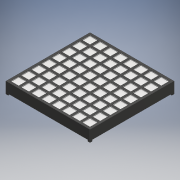
# Autodesk Inventor part: Pieza1
Saved by Autodesk Inventor 2017 (Build 210142000, 142)
## iProperties
Part Number: Pieza1
Material: Genérico
Document SubType Name: Modeling
Designer: Roberto
Density: 1 g/cm^3
Appearance: Valor por defecto
Author: Roberto
Autodesk Inventor part; units mm, degrees
ref_plane "YZ Plane" through (0, 0, 0) normal (1, 0, 0) x (0, 1, 0)
ref_plane "XZ Plane" through (0, 0, 0) normal (0, 1, 0) x (-1, 0, 0)
ref_plane "XY Plane" through (0, 0, 0) normal (0, 0, 1) x (1, 0, 0)
sketch "Boceto1" plane through (0, 0, 0) normal (0, 0, 1) x (1, 0, 0)
  line L0 (0, 0) -> (6, 0)
  line L1 (6, 0) -> (6, 6)
  line L2 (6, 6) -> (0, 6)
  line L3 (0, 6) -> (0, 0)
  constraints: 8 end point
extrude "Extrusión1" add sketch "Boceto1" along normal blind 0.75
sketch "Boceto2" plane through (0, 0, 0.75) normal (0, 0, 1) x (1, 0, 0)
  line L0 (0.1628, 0.7448) -> (0.7447, 0.7448)
  line L1 (0.7447, 0.7448) -> (0.7447, 0.1628)
  line L2 (0.7447, 0.1628) -> (0.1628, 0.1628)
  line L3 (0.1628, 0.1628) -> (0.1628, 0.7448)
  line L4 (0.8902, 0.7448) -> (1.4722, 0.7448)
  line L5 (1.4722, 0.7448) -> (1.4722, 0.1628)
  line L6 (1.4722, 0.1628) -> (0.8902, 0.1628)
  line L7 (0.8902, 0.1628) -> (0.8902, 0.7448)
  line L8 (1.6178, 0.7448) -> (2.1997, 0.7448)
  line L9 (2.1997, 0.7448) -> (2.1997, 0.1628)
  line L10 (2.1997, 0.1628) -> (1.6178, 0.1628)
  line L11 (1.6178, 0.1628) -> (1.6178, 0.7448)
  line L12 (2.3453, 0.7448) -> (2.9273, 0.7448)
  line L13 (2.9273, 0.7448) -> (2.9273, 0.1628)
  line L14 (2.9273, 0.1628) -> (2.3453, 0.1628)
  line L15 (2.3453, 0.1628) -> (2.3453, 0.7448)
  line L16 (3.0727, 0.7448) -> (3.6547, 0.7448)
  line L17 (3.6547, 0.7448) -> (3.6547, 0.1628)
  line L18 (3.6547, 0.1628) -> (3.0727, 0.1628)
  line L19 (3.0727, 0.1628) -> (3.0727, 0.7448)
  line L20 (3.8003, 0.7448) -> (4.3823, 0.7448)
  line L21 (4.3823, 0.7448) -> (4.3823, 0.1628)
  line L22 (4.3823, 0.1628) -> (3.8003, 0.1628)
  line L23 (3.8003, 0.1628) -> (3.8003, 0.7448)
  line L24 (4.5277, 0.7448) -> (5.1097, 0.7448)
  line L25 (5.1097, 0.7448) -> (5.1097, 0.1628)
  line L26 (5.1097, 0.1628) -> (4.5277, 0.1628)
  line L27 (4.5277, 0.1628) -> (4.5277, 0.7448)
  line L28 (5.2553, 0.7448) -> (5.8373, 0.7448)
  line L29 (5.8373, 0.7448) -> (5.8373, 0.1628)
  line L30 (5.8373, 0.1628) -> (5.2553, 0.1628)
  line L31 (5.2553, 0.1628) -> (5.2553, 0.7448)
  line L32 (0, 0) -> (6, 0)
  line L33 (6, 0) -> (6, 6)
  line L34 (6, 6) -> (0, 6)
  line L35 (0, 6) -> (0, 0)
  line L36 (0.1628, 1.4723) -> (0.7447, 1.4723)
  line L37 (0.7447, 1.4723) -> (0.7447, 0.8903)
  line L38 (0.7447, 0.8903) -> (0.1628, 0.8903)
  line L39 (0.1628, 0.8903) -> (0.1628, 1.4723)
  line L40 (0.8902, 1.4723) -> (1.4722, 1.4723)
  line L41 (1.4722, 1.4723) -> (1.4722, 0.8903)
  line L42 (1.4722, 0.8903) -> (0.8902, 0.8903)
  line L43 (0.8902, 0.8903) -> (0.8902, 1.4723)
  line L44 (1.6178, 1.4723) -> (2.1997, 1.4723)
  line L45 (2.1997, 1.4723) -> (2.1997, 0.8903)
  line L46 (2.1997, 0.8903) -> (1.6178, 0.8903)
  line L47 (1.6178, 0.8903) -> (1.6178, 1.4723)
  line L48 (2.3453, 1.4723) -> (2.9273, 1.4723)
  line L49 (2.9273, 1.4723) -> (2.9273, 0.8903)
  line L50 (2.9273, 0.8903) -> (2.3453, 0.8903)
  line L51 (2.3453, 0.8903) -> (2.3453, 1.4723)
  line L52 (3.0727, 1.4723) -> (3.6547, 1.4723)
  line L53 (3.6547, 1.4723) -> (3.6547, 0.8903)
  line L54 (3.6547, 0.8903) -> (3.0727, 0.8903)
  line L55 (3.0727, 0.8903) -> (3.0727, 1.4723)
  line L56 (3.8003, 1.4723) -> (4.3823, 1.4723)
  line L57 (4.3823, 1.4723) -> (4.3823, 0.8903)
  line L58 (4.3823, 0.8903) -> (3.8003, 0.8903)
  line L59 (3.8003, 0.8903) -> (3.8003, 1.4723)
  line L60 (4.5277, 1.4723) -> (5.1097, 1.4723)
  line L61 (5.1097, 1.4723) -> (5.1097, 0.8903)
  line L62 (5.1097, 0.8903) -> (4.5277, 0.8903)
  line L63 (4.5277, 0.8903) -> (4.5277, 1.4723)
  line L64 (5.2553, 1.4723) -> (5.8373, 1.4723)
  line L65 (5.8373, 1.4723) -> (5.8373, 0.8903)
  line L66 (5.8373, 0.8903) -> (5.2553, 0.8903)
  line L67 (5.2553, 0.8903) -> (5.2553, 1.4723)
  line L68 (0.1628, 2.1998) -> (0.7447, 2.1998)
  line L69 (0.7447, 2.1998) -> (0.7447, 1.6178)
  line L70 (0.7447, 1.6178) -> (0.1628, 1.6178)
  line L71 (0.1628, 1.6178) -> (0.1628, 2.1998)
  line L72 (0.8902, 2.1998) -> (1.4722, 2.1998)
  line L73 (1.4722, 2.1998) -> (1.4722, 1.6178)
  line L74 (1.4722, 1.6178) -> (0.8902, 1.6178)
  line L75 (0.8902, 1.6178) -> (0.8902, 2.1998)
  line L76 (1.6178, 2.1998) -> (2.1997, 2.1998)
  line L77 (2.1997, 2.1998) -> (2.1997, 1.6178)
  line L78 (2.1997, 1.6178) -> (1.6178, 1.6178)
  line L79 (1.6178, 1.6178) -> (1.6178, 2.1998)
  line L80 (2.3453, 2.1998) -> (2.9273, 2.1998)
  line L81 (2.9273, 2.1998) -> (2.9273, 1.6178)
  line L82 (2.9273, 1.6178) -> (2.3453, 1.6178)
  line L83 (2.3453, 1.6178) -> (2.3453, 2.1998)
  line L84 (3.0727, 2.1998) -> (3.6547, 2.1998)
  line L85 (3.6547, 2.1998) -> (3.6547, 1.6178)
  line L86 (3.6547, 1.6178) -> (3.0727, 1.6178)
  line L87 (3.0727, 1.6178) -> (3.0727, 2.1998)
  line L88 (3.8003, 2.1998) -> (4.3823, 2.1998)
  line L89 (4.3823, 2.1998) -> (4.3823, 1.6178)
  line L90 (4.3823, 1.6178) -> (3.8003, 1.6178)
  line L91 (3.8003, 1.6178) -> (3.8003, 2.1998)
  line L92 (4.5277, 2.1998) -> (5.1097, 2.1998)
  line L93 (5.1097, 2.1998) -> (5.1097, 1.6178)
  line L94 (5.1097, 1.6178) -> (4.5277, 1.6178)
  line L95 (4.5277, 1.6178) -> (4.5277, 2.1998)
  line L96 (5.2553, 2.1998) -> (5.8373, 2.1998)
  line L97 (5.8373, 2.1998) -> (5.8373, 1.6178)
  line L98 (5.8373, 1.6178) -> (5.2553, 1.6178)
  line L99 (5.2553, 1.6178) -> (5.2553, 2.1998)
  line L100 (0.1628, 2.9273) -> (0.7447, 2.9273)
  line L101 (0.7447, 2.9273) -> (0.7447, 2.3453)
  line L102 (0.7447, 2.3453) -> (0.1628, 2.3453)
  line L103 (0.1628, 2.3453) -> (0.1628, 2.9273)
  line L104 (0.8902, 2.9273) -> (1.4722, 2.9273)
  line L105 (1.4722, 2.9273) -> (1.4722, 2.3453)
  line L106 (1.4722, 2.3453) -> (0.8902, 2.3453)
  line L107 (0.8902, 2.3453) -> (0.8902, 2.9273)
  line L108 (1.6178, 2.9273) -> (2.1997, 2.9273)
  line L109 (2.1997, 2.9273) -> (2.1997, 2.3453)
  line L110 (2.1997, 2.3453) -> (1.6178, 2.3453)
  line L111 (1.6178, 2.3453) -> (1.6178, 2.9273)
  line L112 (2.3453, 2.9273) -> (2.9273, 2.9273)
  line L113 (2.9273, 2.9273) -> (2.9273, 2.3453)
  line L114 (2.9273, 2.3453) -> (2.3453, 2.3453)
  line L115 (2.3453, 2.3453) -> (2.3453, 2.9273)
  line L116 (3.0727, 2.9273) -> (3.6547, 2.9273)
  line L117 (3.6547, 2.9273) -> (3.6547, 2.3453)
  line L118 (3.6547, 2.3453) -> (3.0727, 2.3453)
  line L119 (3.0727, 2.3453) -> (3.0727, 2.9273)
  line L120 (3.8003, 2.9273) -> (4.3823, 2.9273)
  line L121 (4.3823, 2.9273) -> (4.3823, 2.3453)
  line L122 (4.3823, 2.3453) -> (3.8003, 2.3453)
  line L123 (3.8003, 2.3453) -> (3.8003, 2.9273)
  line L124 (4.5277, 2.9273) -> (5.1097, 2.9273)
  line L125 (5.1097, 2.9273) -> (5.1097, 2.3453)
  line L126 (5.1097, 2.3453) -> (4.5277, 2.3453)
  line L127 (4.5277, 2.3453) -> (4.5277, 2.9273)
  line L128 (5.2553, 2.9273) -> (5.8373, 2.9273)
  line L129 (5.8373, 2.9273) -> (5.8373, 2.3453)
  line L130 (5.8373, 2.3453) -> (5.2553, 2.3453)
  line L131 (5.2553, 2.3453) -> (5.2553, 2.9273)
  line L132 (0.1628, 3.6548) -> (0.7447, 3.6548)
  line L133 (0.7447, 3.6548) -> (0.7447, 3.0728)
  line L134 (0.7447, 3.0728) -> (0.1628, 3.0728)
  line L135 (0.1628, 3.0728) -> (0.1628, 3.6548)
  line L136 (0.8902, 3.6548) -> (1.4722, 3.6548)
  line L137 (1.4722, 3.6548) -> (1.4722, 3.0728)
  line L138 (1.4722, 3.0728) -> (0.8902, 3.0728)
  line L139 (0.8902, 3.0728) -> (0.8902, 3.6548)
  line L140 (1.6178, 3.6548) -> (2.1997, 3.6548)
  line L141 (2.1997, 3.6548) -> (2.1997, 3.0728)
  line L142 (2.1997, 3.0728) -> (1.6178, 3.0728)
  line L143 (1.6178, 3.0728) -> (1.6178, 3.6548)
  line L144 (2.3453, 3.6548) -> (2.9273, 3.6548)
  line L145 (2.9273, 3.6548) -> (2.9273, 3.0728)
  line L146 (2.9273, 3.0728) -> (2.3453, 3.0728)
  line L147 (2.3453, 3.0728) -> (2.3453, 3.6548)
  line L148 (3.0727, 3.6548) -> (3.6547, 3.6548)
  line L149 (3.6547, 3.6548) -> (3.6547, 3.0728)
  line L150 (3.6547, 3.0728) -> (3.0727, 3.0728)
  line L151 (3.0727, 3.0728) -> (3.0727, 3.6548)
  line L152 (3.8003, 3.6548) -> (4.3823, 3.6548)
  line L153 (4.3823, 3.6548) -> (4.3823, 3.0728)
  line L154 (4.3823, 3.0728) -> (3.8003, 3.0728)
  line L155 (3.8003, 3.0728) -> (3.8003, 3.6548)
  line L156 (4.5277, 3.6548) -> (5.1097, 3.6548)
  line L157 (5.1097, 3.6548) -> (5.1097, 3.0728)
  line L158 (5.1097, 3.0728) -> (4.5277, 3.0728)
  line L159 (4.5277, 3.0728) -> (4.5277, 3.6548)
  line L160 (5.2553, 3.6548) -> (5.8373, 3.6548)
  line L161 (5.8373, 3.6548) -> (5.8373, 3.0728)
  line L162 (5.8373, 3.0728) -> (5.2553, 3.0728)
  line L163 (5.2553, 3.0728) -> (5.2553, 3.6548)
  line L164 (0.1628, 4.3823) -> (0.7447, 4.3823)
  line L165 (0.7447, 4.3823) -> (0.7447, 3.8003)
  line L166 (0.7447, 3.8003) -> (0.1628, 3.8003)
  line L167 (0.1628, 3.8003) -> (0.1628, 4.3823)
  line L168 (0.8902, 4.3823) -> (1.4722, 4.3823)
  line L169 (1.4722, 4.3823) -> (1.4722, 3.8003)
  line L170 (1.4722, 3.8003) -> (0.8902, 3.8003)
  line L171 (0.8902, 3.8003) -> (0.8902, 4.3823)
  line L172 (1.6178, 4.3823) -> (2.1997, 4.3823)
  line L173 (2.1997, 4.3823) -> (2.1997, 3.8003)
  line L174 (2.1997, 3.8003) -> (1.6178, 3.8003)
  line L175 (1.6178, 3.8003) -> (1.6178, 4.3823)
  line L176 (2.3453, 4.3823) -> (2.9273, 4.3823)
  line L177 (2.9273, 4.3823) -> (2.9273, 3.8003)
  line L178 (2.9273, 3.8003) -> (2.3453, 3.8003)
  line L179 (2.3453, 3.8003) -> (2.3453, 4.3823)
  line L180 (3.0727, 4.3823) -> (3.6547, 4.3823)
  line L181 (3.6547, 4.3823) -> (3.6547, 3.8003)
  line L182 (3.6547, 3.8003) -> (3.0727, 3.8003)
  line L183 (3.0727, 3.8003) -> (3.0727, 4.3823)
  line L184 (3.8003, 4.3823) -> (4.3823, 4.3823)
  line L185 (4.3823, 4.3823) -> (4.3823, 3.8003)
  line L186 (4.3823, 3.8003) -> (3.8003, 3.8003)
  line L187 (3.8003, 3.8003) -> (3.8003, 4.3823)
  line L188 (4.5277, 4.3823) -> (5.1097, 4.3823)
  line L189 (5.1097, 4.3823) -> (5.1097, 3.8003)
  line L190 (5.1097, 3.8003) -> (4.5277, 3.8003)
  line L191 (4.5277, 3.8003) -> (4.5277, 4.3823)
  line L192 (5.2553, 4.3823) -> (5.8373, 4.3823)
  line L193 (5.8373, 4.3823) -> (5.8373, 3.8003)
  line L194 (5.8373, 3.8003) -> (5.2553, 3.8003)
  line L195 (5.2553, 3.8003) -> (5.2553, 4.3823)
  line L196 (0.1628, 5.1098) -> (0.7447, 5.1098)
  line L197 (0.7447, 5.1098) -> (0.7447, 4.5278)
  line L198 (0.7447, 4.5278) -> (0.1628, 4.5278)
  line L199 (0.1628, 4.5278) -> (0.1628, 5.1098)
  line L200 (0.8902, 5.1098) -> (1.4722, 5.1098)
  line L201 (1.4722, 5.1098) -> (1.4722, 4.5278)
  line L202 (1.4722, 4.5278) -> (0.8902, 4.5278)
  line L203 (0.8902, 4.5278) -> (0.8902, 5.1098)
  line L204 (1.6178, 5.1098) -> (2.1997, 5.1098)
  line L205 (2.1997, 5.1098) -> (2.1997, 4.5278)
  line L206 (2.1997, 4.5278) -> (1.6178, 4.5278)
  line L207 (1.6178, 4.5278) -> (1.6178, 5.1098)
  line L208 (2.3453, 5.1098) -> (2.9273, 5.1098)
  line L209 (2.9273, 5.1098) -> (2.9273, 4.5278)
  line L210 (2.9273, 4.5278) -> (2.3453, 4.5278)
  line L211 (2.3453, 4.5278) -> (2.3453, 5.1098)
  line L212 (3.0727, 5.1098) -> (3.6547, 5.1098)
  line L213 (3.6547, 5.1098) -> (3.6547, 4.5278)
  line L214 (3.6547, 4.5278) -> (3.0727, 4.5278)
  line L215 (3.0727, 4.5278) -> (3.0727, 5.1098)
  line L216 (3.8003, 5.1098) -> (4.3823, 5.1098)
  line L217 (4.3823, 5.1098) -> (4.3823, 4.5278)
  line L218 (4.3823, 4.5278) -> (3.8003, 4.5278)
  line L219 (3.8003, 4.5278) -> (3.8003, 5.1098)
  line L220 (4.5277, 5.1098) -> (5.1097, 5.1098)
  line L221 (5.1097, 5.1098) -> (5.1097, 4.5278)
  line L222 (5.1097, 4.5278) -> (4.5277, 4.5278)
  line L223 (4.5277, 4.5278) -> (4.5277, 5.1098)
  line L224 (5.2553, 5.1098) -> (5.8373, 5.1098)
  line L225 (5.8373, 5.1098) -> (5.8373, 4.5278)
  line L226 (5.8373, 4.5278) -> (5.2553, 4.5278)
  line L227 (5.2553, 4.5278) -> (5.2553, 5.1098)
  line L228 (0.1628, 5.8373) -> (0.7447, 5.8373)
  line L229 (0.7447, 5.8373) -> (0.7447, 5.2553)
  line L230 (0.7447, 5.2553) -> (0.1628, 5.2553)
  line L231 (0.1628, 5.2553) -> (0.1628, 5.8373)
  line L232 (0.8902, 5.8373) -> (1.4722, 5.8373)
  line L233 (1.4722, 5.8373) -> (1.4722, 5.2553)
  line L234 (1.4722, 5.2553) -> (0.8902, 5.2553)
  line L235 (0.8902, 5.2553) -> (0.8902, 5.8373)
  line L236 (1.6178, 5.8373) -> (2.1997, 5.8373)
  line L237 (2.1997, 5.8373) -> (2.1997, 5.2553)
  line L238 (2.1997, 5.2553) -> (1.6178, 5.2553)
  line L239 (1.6178, 5.2553) -> (1.6178, 5.8373)
  line L240 (2.3453, 5.8373) -> (2.9273, 5.8373)
  line L241 (2.9273, 5.8373) -> (2.9273, 5.2553)
  line L242 (2.9273, 5.2553) -> (2.3453, 5.2553)
  line L243 (2.3453, 5.2553) -> (2.3453, 5.8373)
  line L244 (3.0727, 5.8373) -> (3.6547, 5.8373)
  line L245 (3.6547, 5.8373) -> (3.6547, 5.2553)
  line L246 (3.6547, 5.2553) -> (3.0727, 5.2553)
  line L247 (3.0727, 5.2553) -> (3.0727, 5.8373)
  line L248 (3.8003, 5.8373) -> (4.3823, 5.8373)
  line L249 (4.3823, 5.8373) -> (4.3823, 5.2553)
  line L250 (4.3823, 5.2553) -> (3.8003, 5.2553)
  line L251 (3.8003, 5.2553) -> (3.8003, 5.8373)
  line L252 (4.5277, 5.8373) -> (5.1097, 5.8373)
  line L253 (5.1097, 5.8373) -> (5.1097, 5.2553)
  line L254 (5.1097, 5.2553) -> (4.5277, 5.2553)
  line L255 (4.5277, 5.2553) -> (4.5277, 5.8373)
  line L256 (5.2553, 5.8373) -> (5.8373, 5.8373)
  line L257 (5.8373, 5.8373) -> (5.8373, 5.2553)
  line L258 (5.8373, 5.2553) -> (5.2553, 5.2553)
  line L259 (5.2553, 5.2553) -> (5.2553, 5.8373)
  constraints: 520 end point
extrude "Extrusión2" add sketch "Boceto2" along normal blind 0.05
sketch "Boceto3" plane through (0, 0, 0) normal (0, 0, -1) x (-1, 0, 0)
  line L0 (-5.8373, 5.8373) -> (-0.1628, 5.8373)
  line L1 (-0.1628, 5.8373) -> (-0.1628, 0.1628)
  line L2 (-0.1628, 0.1628) -> (-5.8373, 0.1628)
  line L3 (-5.8373, 0.1628) -> (-5.8373, 5.8373)
  line L4 (-5.2553, 5.8373) -> (-5.8373, 5.8373) projected
  line L5 (-0.1628, 5.8373) -> (-0.1628, 5.2553) projected
  line L6 (-0.1628, 0.1628) -> (-0.7447, 0.1628) projected
  line L7 (-5.8373, 0.1628) -> (-5.2553, 0.1628) projected
  line L8 (-5.8373, 0.1628) -> (-0.1628, 0.1628)
  line L9 (-0.1628, 0.1628) -> (-0.1628, 5.8373)
  line L10 (-0.1628, 5.8373) -> (-5.8373, 5.8373)
  line L11 (-5.8373, 5.2553) -> (-5.8373, 5.8373) projected
  line L12 (-5.8373, 0.1628) -> (-5.8373, 5.8373)
  constraints: 16 end point, 2 horizontal
extrude "Extrusión3" cut sketch "Boceto3" against normal blind 0.2
sketch "Boceto4" plane through (0, 0, 0) normal (0, 0, -1) x (-1, 0, 0)
  line L0 (-5.8373, 0.1628) -> (-5.8373, 5.8373) projected
  line L1 (-5.8373, 5.8373) -> (-0.1628, 5.8373) projected
  line L2 (-0.1628, 5.8373) -> (-0.1628, 0.1628) projected
  line L3 (-0.1628, 0.1628) -> (-5.8373, 0.1628) projected
  line L4 (0, 0) -> (-6, 0) projected
  line L5 (0, 6) -> (0, 0) projected
  line L6 (-6, 6) -> (0, 6) projected
  line L7 (-6, 0) -> (-6, 6) projected
  line L8 (-0.1628, 0) -> (-0.1628, 0.1628)
  line L9 (-0.1628, 0.1628) -> (0, 0.1628)
  line L10 (-0.1628, 5.8373) -> (0, 5.8373)
  line L11 (-0.1628, 6) -> (-0.1628, 5.8373)
  line L12 (-5.2553, 5.8373) -> (-5.8373, 5.8373) projected
  line L13 (-5.8373, 5.8373) -> (-6, 5.8373)
  line L14 (-5.8373, 6) -> (-5.8373, 5.8373)
  line L15 (-5.8373, 0.1628) -> (-6, 0.1628)
  line L16 (-5.8373, 0) -> (-5.8373, 0.1628)
  line L17 (-5.8373, 0.1628) -> (-5.8373, 5.8373) projected
  line L18 (-5.8373, 0.1628) -> (-0.1628, 0.1628)
  line L19 (-0.1628, 0.1628) -> (-0.1628, 0)
  line L20 (-0.1628, 0) -> (-5.8373, 0)
  line L21 (-5.8373, 0) -> (-5.8373, 0.1628)
  line L22 (-0.1628, 0.1628) -> (0, 0.1628)
  line L23 (0, 0.1628) -> (0, 5.8373)
  line L24 (0, 5.8373) -> (-0.1628, 5.8373)
  line L25 (-0.1628, 5.8373) -> (-0.1628, 0.1628)
  line L26 (-0.1628, 6) -> (-5.8373, 6)
  line L27 (-5.8373, 6) -> (-5.8373, 5.8373)
  line L28 (-5.8373, 5.8373) -> (-0.1628, 5.8373)
  line L29 (-0.1628, 5.8373) -> (-0.1628, 6)
  line L30 (-5.8373, 5.8373) -> (-6, 5.8373)
  line L31 (-6, 5.8373) -> (-6, 0.1628)
  line L32 (-6, 0.1628) -> (-5.8373, 0.1628)
  line L33 (-5.8373, 0.1628) -> (-5.8373, 5.8373)
  constraints: 48 end point, 8 parallel, 7 horizontal, 4 perpendicular
extrude "Extrusión4" cut sketch "Boceto4" against normal blind 0.1 contours L15 L7 L13 L0 | L3 L8 L4 L16 | L14 L6 L11 L1 | L2 L10 L5 L9
sketch "Boceto5" plane through (0, 0, 0.2) normal (0, 0, -1) x (-1, 0, 0)
  line L0 (-6, 0) -> (0, 0)
  line L1 (0, 0) -> (0, 6)
  line L2 (0, 6) -> (-6, 6)
  line L3 (-6, 6) -> (-6, 0)
  line L4 (-6, 0) -> (0, 0)
  line L5 (0, 6) -> (0, 4.5)
  circle A0 centre (-1.5, 4.5) radius 0.085
  circle A1 centre (-1.5, 1.5) radius 0.085
  circle A2 centre (-4.5, 4.5) radius 0.085
  circle A3 centre (-4.5, 1.5) radius 0.085
  line L6 (0, 6) -> (-1, 6)
  line L7 (-1, 5.4) -> (-1, 5.15)
  line L8 (-1, 5.15) -> (-4.95, 5.15)
  line L9 (-4.95, 5.15) -> (-4.95, 5.4)
  line L10 (-4.95, 5.4) -> (-1, 5.4)
  line L11 (-1, 0.6) -> (-1, 0.85)
  line L12 (-1, 0.85) -> (-4.95, 0.85)
  line L13 (-4.95, 0.85) -> (-4.95, 0.6)
  line L14 (-4.95, 0.6) -> (-1, 0.6)
  line L15 (-6, 4.8) -> (0, 4.8)
  line L16 (-6, 1.2) -> (0, 1.2)
  line L17 (-6, 5.65) -> (0, 5.65)
  line L18 (-6, 0.35) -> (0, 0.35)
  line L19 (-6, 4.8) -> (-6, 3.6)
  point P0 (0, 0)
  constraints: 40 end point, 13 point on line, 4 centre point
extrude "Extrusión5" cut sketch "Boceto5" against normal blind 0.3 contours A0 | A1 | A2 | A3
sketch "Boceto6" plane through (0, 0, 0.2) normal (0, 0, -1) x (-1, 0, 0)
  line L0 (-6, 0) -> (0, 0)
  line L1 (0, 0) -> (0, 6)
  line L2 (0, 6) -> (-6, 6)
  line L3 (-6, 6) -> (-6, 0)
  line L4 (-6, 0) -> (0, 0)
  line L5 (0, 6) -> (0, 4.5)
  circle A0 centre (-1.5, 4.5) radius 0.085
  circle A1 centre (-1.5, 1.5) radius 0.085
  circle A2 centre (-4.5, 4.5) radius 0.085
  circle A3 centre (-4.5, 1.5) radius 0.085
  line L6 (0, 6) -> (-1, 6)
  line L7 (-1, 5.4) -> (-1, 5.15)
  line L8 (-1, 5.15) -> (-4.95, 5.15)
  line L9 (-4.95, 5.15) -> (-4.95, 5.4)
  line L10 (-4.95, 5.4) -> (-1, 5.4)
  line L11 (-1, 0.6) -> (-1, 0.85)
  line L12 (-1, 0.85) -> (-4.95, 0.85)
  line L13 (-4.95, 0.85) -> (-4.95, 0.6)
  line L14 (-4.95, 0.6) -> (-1, 0.6)
  line L15 (-6, 4.8) -> (0, 4.8)
  line L16 (-6, 1.2) -> (0, 1.2)
  line L17 (-6, 5.65) -> (0, 5.65)
  line L18 (-6, 0.35) -> (0, 0.35)
  line L19 (-6, 4.8) -> (-6, 3.6)
  point P0 (0, 0)
  point P1 (0, 0)
  constraints: 40 end point, 13 point on line, 4 centre point
extrude "Extrusión6" add sketch "Boceto6" along normal blind 0.5 contours L7 L8 L9 L10 | L14 L13 L12 L11
